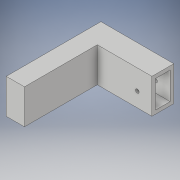
# Autodesk Inventor part: hollowPart
Saved by Autodesk Inventor 2019 (Build 230136000, 136)
## iProperties
Created: 2018-11-15
Part Number: hollowPart
Material: Generic
Document SubType Name: Modeling
Designer: Charlie
Density: 1 g/cm^3
Appearance: Default
Author: Charlie
Autodesk Inventor part; units mm, degrees
ref_plane "YZ Plane" through (0, 0, 0) normal (1, 0, 0) x (0, 1, 0)
ref_plane "XZ Plane" through (0, 0, 0) normal (0, 1, 0) x (-1, 0, 0)
ref_plane "XY Plane" through (0, 0, 0) normal (0, 0, 1) x (1, 0, 0)
sketch "Sketch1" plane through (0, 0, 0) normal (0, 0, 1) x (1, 0, 0)
  line L0 (-17.78, 6.35) -> (7.62, 6.35)
  line L1 (7.62, 6.35) -> (7.62, -5.715)
  line L2 (7.62, -5.715) -> (-17.78, -5.715)
  line L3 (-17.78, -5.715) -> (-17.78, 6.35)
  point P0 (0, 0)
  dimension "d0" = 25.4
  dimension "d1" = 12.065
  dimension "d2" = 7.62
  dimension "d3" = 6.35
  constraints: 8 end point, 2 parallel, 1 horizontal, 1 perpendicular
  measures "d0" distance of L1.end L2.end
  measures "d1" distance between parallel lines of L2 L0
  measures "d2" distance from line of L1 point (0, 0)
  measures "d3" distance from line of L0 point (0, 0)
extrude "Extrusion1" add sketch "Sketch1" along normal blind 7.62
sketch "Sketch2" plane through (7.62, -5.715, 0) normal (1, 0, 0) x (0, 0, -1)
  line L0 (-6.35, 10.795) -> (-1.27, 10.795)
  line L1 (-1.27, 10.795) -> (-1.27, 1.27)
  line L2 (-1.27, 1.27) -> (-6.35, 1.27)
  line L3 (-6.35, 1.27) -> (-6.35, 10.795)
  line L4 (-7.62, 0) -> (-7.62, 12.065) projected
  line L5 (0, 12.065) -> (-7.62, 12.065) projected
  line L6 (0, 12.065) -> (0, 0) projected
  line L7 (0, 0) -> (-7.62, 0) projected
  point P0 (0, 5.715)
  dimension "d8" = 1.27
  dimension "d9" = 1.27
  dimension "d23" = 1.27
  dimension "d24" = 1.27
  constraints: 8 end point, 2 parallel, 1 horizontal, 1 perpendicular
  measures "d8" distance between parallel lines of L4 L3
  measures "d9" distance between parallel lines of L5 L0
  measures "d23" distance between parallel lines of L6 L1
  measures "d24" distance between parallel lines of L7 L2
extrude "Extrusion2" cut sketch "Sketch2" against normal blind 21.59 contours L0 L1 L2 L3
sketch "Sketch3" plane through (0, 0, 7.62) normal (0, 0, 1) x (1, 0, 0)
  line L0 (-17.78, 6.35) -> (-17.78, -5.715) projected
  line L1 (7.62, 6.35) -> (-17.78, 6.35) projected
  line L2 (-17.78, -5.715) -> (7.62, -5.715) projected
  line L3 (-17.78, 6.35) -> (-11.43, 6.35)
  line L4 (-11.43, 6.35) -> (-11.43, -5.715)
  line L5 (-11.43, -5.715) -> (-17.78, -5.715)
  line L6 (-17.78, -5.715) -> (-17.78, 6.35)
  point P0 (0, 0)
  dimension "d26" = 6.35
  constraints: 8 end point, 2 parallel, 1 horizontal, 1 perpendicular, 1 point on line
  measures "d26" distance of L4.end L5.end
extrude "Extrusion3" add sketch "Sketch3" along normal blind 25.4
sketch "Sketch4" plane through (0, 0, 7.62) normal (0, 0, 1) x (1, 0, 0)
  circle A0 centre (2.54, -0.635) radius 0.635
  line L0 (7.62, 6.35) -> (-17.78, 6.35) projected
  point P0 (0, 0)
  point P1 (-11.43, 6.35)
  dimension "d18" = 1.27
  dimension "d20" = 6.985
  dimension "d25" = 2.54
  constraints: 1 centre point
  measures "d18" diameter of A0
  measures "d20" distance from line of L0 A0.centre
  measures "d25" horizontal distance of A0.centre point (0, 0)
extrude "Extrusion4" cut sketch "Sketch4" against normal blind 50.8
body "Solid1"
